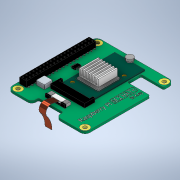
# Autodesk Inventor part: Raspberry Pi HAT+
Saved by Autodesk Inventor 2021 (Build 250183000, 183)
## iProperties
Created: 2025-01-26
Part Number: Raspberry Pi HAT+
Material: Generic
Document SubType Name: Modeling
Designer: 22liatho
Density: 1 g/cm^3
Appearance: Default
Author: 22liatho
Autodesk Inventor part; units mm, degrees
(part 1 of 2)
sketch "Sketch1" plane through (0, 0, 0) normal (0, 1, 0) x (-1, 0, 0)
  line L0 (-53, -65) -> (-3.5, -65)
  line L1 (0, -61.5) -> (0, -3.5)
  arc A0 (-3.5, -65) -> (0, -61.5) centre (-3.5, -61.5) ccw
  arc A1 (0, -3.5) -> (-3.5, 0) centre (-3.5, -3.5) ccw
  arc A2 (-53, 0) -> (-56.5, -3.5) centre (-53, -3.5) ccw
  arc A3 (-56.5, -61.5) -> (-53, -65) centre (-53, -61.5) ccw
  line L2 (-56.5, -57.5) -> (-40, -57.5)
  line L3 (-40, -57.5) -> (-40, -47.5)
  line L4 (-40, -47.5) -> (-56.5, -47.5)
  circle A4 centre (-53, -3.5) radius 3
  line L5 (-17.5, 0) -> (-17.5, -5)
  line L6 (-17.5, -5) -> (-35.5, -5)
  line L7 (-35.5, -5) -> (-35.5, 0)
  line L8 (-1.5, -7.1) -> (-6.5, -7.1)
  line L9 (-6.5, -7.1) -> (-6.5, -57.9)
  line L10 (-6.5, -57.9) -> (-1.5, -57.9)
  line L11 (-1.5, -57.9) -> (-1.5, -7.1)
  line L12 (-3.5, 0) -> (-17.5, 0)
  line L13 (-35.5, 0) -> (-53, 0)
  line L14 (-56.5, -3.5) -> (-56.5, -47.5)
  line L15 (-56.5, -57.5) -> (-56.5, -61.5)
  circle A5 centre (-53, -61.5) radius 3
  circle A6 centre (-53, -3.5) radius 1.375
  circle A7 centre (-53, -61.5) radius 1.375
  circle A8 centre (-4, -61.5) radius 3
  circle A9 centre (-4, -61.5) radius 1.375
  circle A10 centre (-4, -3.5) radius 3
  circle A11 centre (-4, -3.5) radius 1.375
  line L16 (-1.5, -32.5) -> (-6.5, -32.5) construction
  point P0 (0, 0)
  point P1 (-56.5, -65)
  point P2 (0, -65)
  point P3 (-4, -32.5)
  dimension "d82" = 3
  dimension "d83" = 3
  dimension "d2" = 3.5
  dimension "d5" = 7.5
  dimension "d6" = 10
  dimension "d10" = 18
  dimension "d12" = 17.5
  dimension "d17" = 5
  dimension "d18" = 56.5
  dimension "d19" = 16.5
  dimension "d20" = 65
  dimension "d21" = 3.5
  dimension "d22" = 3.5
  dimension "d23" = 58
  dimension "d24" = 3.5
  dimension "d25" = 6
  dimension "d26" = 6
  dimension "d27" = 2.75
  dimension "d28" = 2.75
  dimension "d29" = 3.5
  dimension "d31" = 6
  dimension "d32" = 2.75
  dimension "d35" = 49
  dimension "d36" = 6
  dimension "d37" = 49
  dimension "d38" = 3.5
  dimension "d39" = 2.75
  dimension "d40" = 29
  dimension "d43" = 5
  dimension "d44" = 56.5
  dimension "d206" = 50.8
  constraints: 34 end point, 12 centre point, 12 tangent, 10 perpendicular, 8 point on circle, 6 parallel, 5 horizontal, 4 coincident, 4 point on line, 3 equal radius, 3 midpoint, 1 horizontal alignment, 1 vertical, 1 vertical alignment
  measures "d2" radius of A0
  measures "d5" distance between parallel lines of L0 L2
  measures "d6" distance between parallel lines of L2 L4
  measures "d10" distance between parallel lines of L7 L5
  measures "d12" distance between parallel lines of L1 L5
  measures "d17" distance between parallel lines of L12 L6
  measures "d18" distance between parallel lines of L1 L14
  measures "d19" distance between parallel lines of L14 L3
  measures "d20" distance between parallel lines of L13 L0
  measures "d21" distance from line of L14 A4.centre
  measures "d22" distance from line of L13 A4.centre
  measures "d23" distance of A2.centre A5.centre
  measures "d24" distance from line of L15 A5.centre
  measures "d25" diameter of A4
  measures "d26" diameter of A5
  measures "d27" diameter of A6
  measures "d28" diameter of A7
  measures "d29" distance from line of L0 A8.centre
  measures "d31" diameter of A8
  measures "d32" diameter of A9
  measures "d35" distance of A5.centre A8.centre
  measures "d36" diameter of A10
  measures "d37" distance of A4.centre A10.centre
  measures "d38" distance from line of L12 A10.centre
  measures "d39" diameter of A11
  measures "d40" distance from line of A10.centre L16
  measures "d43" distance between parallel lines of L11 L9
  measures "d44" distance from line of point (-56.5, -65) L1
  measures "d206" distance of L10.end L8.start
extrude "Extrusion1" add sketch "Sketch1" along normal blind 1.6 contours A3 L15 L2 L3 L4 L14 A2 L13 L7 L6 L5 L12 A1 L1 A0 L0 | L11 L10 L9 L8
extrude "Extrusion2" add sketch "Sketch1" along normal blind 1.58 contours A4 | A5 | A8 | A10
extrude "Extrusion3" add sketch "Sketch1" along normal blind 5.88 contours L11 L10 L9 L8
fillet "Fillet1" radius 3 2 edges at (35.5, 0.8, 0) (17.5, 0.8, 0)
sketch "Sketch2" plane through (0, 5.88, 0) normal (0, 1, 0) x (1, 0, 0)
  line L0 (2.45, 8.69) -> (3.09, 8.69)
  line L1 (3.09, 8.69) -> (3.09, 8.05)
  line L2 (3.09, 8.05) -> (2.45, 8.05)
  line L3 (2.45, 8.05) -> (2.45, 8.69)
  line L4 (1.5, 57.9) -> (1.5, 7.1) projected
  line L5 (1.5, 7.1) -> (6.5, 7.1) projected
  line L6 (5.55, 8.69) -> (5.55, 8.05)
  line L7 (5.55, 8.05) -> (4.91, 8.05)
  line L8 (4.91, 8.05) -> (4.91, 8.69)
  line L9 (4.91, 8.69) -> (5.55, 8.69)
  line L10 (3.09, 11.23) -> (3.09, 10.59)
  line L11 (3.09, 10.59) -> (2.45, 10.59)
  line L12 (2.45, 10.59) -> (2.45, 11.23)
  line L13 (2.45, 11.23) -> (3.09, 11.23)
  line L14 (5.55, 11.23) -> (5.55, 10.59)
  line L15 (5.55, 10.59) -> (4.91, 10.59)
  line L16 (4.91, 10.59) -> (4.91, 11.23)
  line L17 (4.91, 11.23) -> (5.55, 11.23)
  line L18 (3.09, 13.77) -> (3.09, 13.13)
  line L19 (3.09, 13.13) -> (2.45, 13.13)
  line L20 (2.45, 13.13) -> (2.45, 13.77)
  line L21 (2.45, 13.77) -> (3.09, 13.77)
  line L22 (5.55, 13.77) -> (5.55, 13.13)
  line L23 (5.55, 13.13) -> (4.91, 13.13)
  line L24 (4.91, 13.13) -> (4.91, 13.77)
  line L25 (4.91, 13.77) -> (5.55, 13.77)
  line L26 (3.09, 16.31) -> (3.09, 15.67)
  line L27 (3.09, 15.67) -> (2.45, 15.67)
  line L28 (2.45, 15.67) -> (2.45, 16.31)
  line L29 (2.45, 16.31) -> (3.09, 16.31)
  line L30 (5.55, 16.31) -> (5.55, 15.67)
  line L31 (5.55, 15.67) -> (4.91, 15.67)
  line L32 (4.91, 15.67) -> (4.91, 16.31)
  line L33 (4.91, 16.31) -> (5.55, 16.31)
  line L34 (3.09, 18.85) -> (3.09, 18.21)
  line L35 (3.09, 18.21) -> (2.45, 18.21)
  line L36 (2.45, 18.21) -> (2.45, 18.85)
  line L37 (2.45, 18.85) -> (3.09, 18.85)
  line L38 (5.55, 18.85) -> (5.55, 18.21)
  line L39 (5.55, 18.21) -> (4.91, 18.21)
  line L40 (4.91, 18.21) -> (4.91, 18.85)
  line L41 (4.91, 18.85) -> (5.55, 18.85)
  line L42 (3.09, 21.39) -> (3.09, 20.75)
  line L43 (3.09, 20.75) -> (2.45, 20.75)
  line L44 (2.45, 20.75) -> (2.45, 21.39)
  line L45 (2.45, 21.39) -> (3.09, 21.39)
  line L46 (5.55, 21.39) -> (5.55, 20.75)
  line L47 (5.55, 20.75) -> (4.91, 20.75)
  line L48 (4.91, 20.75) -> (4.91, 21.39)
  line L49 (4.91, 21.39) -> (5.55, 21.39)
  line L50 (3.09, 23.93) -> (3.09, 23.29)
  line L51 (3.09, 23.29) -> (2.45, 23.29)
  line L52 (2.45, 23.29) -> (2.45, 23.93)
  line L53 (2.45, 23.93) -> (3.09, 23.93)
  line L54 (5.55, 23.93) -> (5.55, 23.29)
  line L55 (5.55, 23.29) -> (4.91, 23.29)
  line L56 (4.91, 23.29) -> (4.91, 23.93)
  line L57 (4.91, 23.93) -> (5.55, 23.93)
  line L58 (3.09, 26.47) -> (3.09, 25.83)
  line L59 (3.09, 25.83) -> (2.45, 25.83)
  line L60 (2.45, 25.83) -> (2.45, 26.47)
  line L61 (2.45, 26.47) -> (3.09, 26.47)
  line L62 (5.55, 26.47) -> (5.55, 25.83)
  line L63 (5.55, 25.83) -> (4.91, 25.83)
  line L64 (4.91, 25.83) -> (4.91, 26.47)
  line L65 (4.91, 26.47) -> (5.55, 26.47)
  line L66 (3.09, 29.01) -> (3.09, 28.37)
  line L67 (3.09, 28.37) -> (2.45, 28.37)
  line L68 (2.45, 28.37) -> (2.45, 29.01)
  line L69 (2.45, 29.01) -> (3.09, 29.01)
  line L70 (5.55, 29.01) -> (5.55, 28.37)
  line L71 (5.55, 28.37) -> (4.91, 28.37)
  line L72 (4.91, 28.37) -> (4.91, 29.01)
  line L73 (4.91, 29.01) -> (5.55, 29.01)
  line L74 (3.09, 31.55) -> (3.09, 30.91)
  line L75 (3.09, 30.91) -> (2.45, 30.91)
  line L76 (2.45, 30.91) -> (2.45, 31.55)
  line L77 (2.45, 31.55) -> (3.09, 31.55)
  line L78 (5.55, 31.55) -> (5.55, 30.91)
  line L79 (5.55, 30.91) -> (4.91, 30.91)
  line L80 (4.91, 30.91) -> (4.91, 31.55)
  line L81 (4.91, 31.55) -> (5.55, 31.55)
  line L82 (3.09, 34.09) -> (3.09, 33.45)
  line L83 (3.09, 33.45) -> (2.45, 33.45)
  line L84 (2.45, 33.45) -> (2.45, 34.09)
  line L85 (2.45, 34.09) -> (3.09, 34.09)
  line L86 (5.55, 34.09) -> (5.55, 33.45)
  line L87 (5.55, 33.45) -> (4.91, 33.45)
  line L88 (4.91, 33.45) -> (4.91, 34.09)
  line L89 (4.91, 34.09) -> (5.55, 34.09)
  line L90 (3.09, 36.63) -> (3.09, 35.99)
  line L91 (3.09, 35.99) -> (2.45, 35.99)
  line L92 (2.45, 35.99) -> (2.45, 36.63)
  line L93 (2.45, 36.63) -> (3.09, 36.63)
  line L94 (5.55, 36.63) -> (5.55, 35.99)
  line L95 (5.55, 35.99) -> (4.91, 35.99)
  line L96 (4.91, 35.99) -> (4.91, 36.63)
  line L97 (4.91, 36.63) -> (5.55, 36.63)
  line L98 (3.09, 39.17) -> (3.09, 38.53)
  line L99 (3.09, 38.53) -> (2.45, 38.53)
  line L100 (2.45, 38.53) -> (2.45, 39.17)
  line L101 (2.45, 39.17) -> (3.09, 39.17)
  line L102 (5.55, 39.17) -> (5.55, 38.53)
  line L103 (5.55, 38.53) -> (4.91, 38.53)
  line L104 (4.91, 38.53) -> (4.91, 39.17)
  line L105 (4.91, 39.17) -> (5.55, 39.17)
  line L106 (3.09, 41.71) -> (3.09, 41.07)
  line L107 (3.09, 41.07) -> (2.45, 41.07)
  line L108 (2.45, 41.07) -> (2.45, 41.71)
  line L109 (2.45, 41.71) -> (3.09, 41.71)
  line L110 (5.55, 41.71) -> (5.55, 41.07)
  line L111 (5.55, 41.07) -> (4.91, 41.07)
  line L112 (4.91, 41.07) -> (4.91, 41.71)
  line L113 (4.91, 41.71) -> (5.55, 41.71)
  line L114 (3.09, 44.25) -> (3.09, 43.61)
  line L115 (3.09, 43.61) -> (2.45, 43.61)
  line L116 (2.45, 43.61) -> (2.45, 44.25)
  line L117 (2.45, 44.25) -> (3.09, 44.25)
  line L118 (5.55, 44.25) -> (5.55, 43.61)
  line L119 (5.55, 43.61) -> (4.91, 43.61)
  line L120 (4.91, 43.61) -> (4.91, 44.25)
  line L121 (4.91, 44.25) -> (5.55, 44.25)
  line L122 (3.09, 46.79) -> (3.09, 46.15)
  line L123 (3.09, 46.15) -> (2.45, 46.15)
  line L124 (2.45, 46.15) -> (2.45, 46.79)
  line L125 (2.45, 46.79) -> (3.09, 46.79)
  line L126 (5.55, 46.79) -> (5.55, 46.15)
  line L127 (5.55, 46.15) -> (4.91, 46.15)
  line L128 (4.91, 46.15) -> (4.91, 46.79)
  line L129 (4.91, 46.79) -> (5.55, 46.79)
  line L130 (3.09, 49.33) -> (3.09, 48.69)
  line L131 (3.09, 48.69) -> (2.45, 48.69)
  line L132 (2.45, 48.69) -> (2.45, 49.33)
  line L133 (2.45, 49.33) -> (3.09, 49.33)
  line L134 (5.55, 49.33) -> (5.55, 48.69)
  line L135 (5.55, 48.69) -> (4.91, 48.69)
  line L136 (4.91, 48.69) -> (4.91, 49.33)
  line L137 (4.91, 49.33) -> (5.55, 49.33)
  line L138 (3.09, 51.87) -> (3.09, 51.23)
  line L139 (3.09, 51.23) -> (2.45, 51.23)
  line L140 (2.45, 51.23) -> (2.45, 51.87)
  line L141 (2.45, 51.87) -> (3.09, 51.87)
  line L142 (5.55, 51.87) -> (5.55, 51.23)
  line L143 (5.55, 51.23) -> (4.91, 51.23)
  line L144 (4.91, 51.23) -> (4.91, 51.87)
  line L145 (4.91, 51.87) -> (5.55, 51.87)
  line L146 (3.09, 54.41) -> (3.09, 53.77)
  line L147 (3.09, 53.77) -> (2.45, 53.77)
  line L148 (2.45, 53.77) -> (2.45, 54.41)
  line L149 (2.45, 54.41) -> (3.09, 54.41)
  line L150 (5.55, 54.41) -> (5.55, 53.77)
  line L151 (5.55, 53.77) -> (4.91, 53.77)
  line L152 (4.91, 53.77) -> (4.91, 54.41)
  line L153 (4.91, 54.41) -> (5.55, 54.41)
  line L154 (3.09, 56.95) -> (3.09, 56.31)
  line L155 (3.09, 56.31) -> (2.45, 56.31)
  line L156 (2.45, 56.31) -> (2.45, 56.95)
  line L157 (2.45, 56.95) -> (3.09, 56.95)
  line L158 (5.55, 56.95) -> (5.55, 56.31)
  line L159 (5.55, 56.31) -> (4.91, 56.31)
  line L160 (4.91, 56.31) -> (4.91, 56.95)
  line L161 (4.91, 56.95) -> (5.55, 56.95)
  line L162 (6.5, 57.9) -> (1.5, 57.9) projected
  point P0 (0, 0)
  dimension "d54" = 0.95
  dimension "d55" = 0.95
  dimension "d56" = 0.64
  dimension "d57" = 0.64
  dimension "d60" = 2.46
  dimension "d63" = 2.54
  dimension "d66" = 0.95
  constraints: 320 end point, 2 horizontal, 2 parallel, 1 perpendicular, 1 vertical, 312 other
  measures "d54" distance between parallel lines of L4 L3
  measures "d55" distance between parallel lines of L5 L2
  measures "d56" distance of L0.start L0.end
  measures "d57" distance of L0.end L1.end
  measures "d60" distance of L0.end L6.start
  measures "d63" distance of L0.end L10.start
  measures "d66" distance between parallel lines of L162 L157
extrude "Extrusion4" cut sketch "Sketch2" against normal blind 1
fillet "Fillet4" radius 1 6 edges at (40, 0.8, -57.5) (40, 0.8, -47.5) (56.5, 0.8, -47.5) (56.5, 0.8, -57.5) (17.5, 0.8, -5) (35.5, 0.8, -5)
sketch "Sketch3" plane through (0, 1.6, 0) normal (0, 1, 0) x (1, 0, 0)
  line L0 (17.25, 19) -> (39.25, 19)
  line L1 (39.25, 19) -> (39.25, 61)
  line L2 (39.25, 61) -> (17.25, 61)
  line L3 (17.25, 61) -> (17.25, 19)
  circle A0 centre (35.75, 49.5) radius 1.25
  circle A1 centre (20.75, 26.5) radius 1.25
  line L4 (53, 65) -> (3.5, 65) projected
  circle A2 centre (28.25, 61) radius 2
  line L5 (19.75, 29.5) -> (36.75, 29.5)
  line L6 (36.75, 29.5) -> (36.75, 46.5)
  line L7 (36.75, 46.5) -> (19.75, 46.5)
  line L8 (19.75, 46.5) -> (19.75, 29.5)
  line L9 (18.25, 19) -> (18.25, 22.5)
  line L10 (21.75, 19) -> (21.75, 22)
  arc A3 (22.75, 22) -> (21.75, 22) centre (22.25, 22) ccw
  line L11 (22.75, 22) -> (22.75, 19)
  line L12 (33.75, 19) -> (33.75, 22)
  arc A4 (34.75, 22) -> (33.75, 22) centre (34.25, 22) ccw
  line L13 (34.75, 22) -> (34.75, 19)
  line L14 (38.25, 19) -> (38.25, 22.5)
  line L15 (39.25, 23) -> (38.75, 23)
  arc A5 (38.75, 23) -> (38.25, 22.5) centre (38.75, 22.5) ccw
  line L16 (17.25, 23) -> (17.75, 23)
  arc A6 (18.25, 22.5) -> (17.75, 23) centre (17.75, 22.5) ccw
  point P0 (0, 0)
  point P1 (28.25, 65)
  point P2 (28.25, 46.5)
  point P3 (34.25, 22.5)
  point P4 (22.25, 22.5)
  point P5 (30.25, 61)
  point P6 (26.25, 61)
  dimension "d69" = 22
  dimension "d70" = 42
  dimension "d71" = 2.5
  dimension "d72" = 2.5
  dimension "d73" = 18.5
  dimension "d74" = 3.5
  dimension "d75" = 30.5
  dimension "d76" = 7.5
  dimension "d78" = 4
  dimension "d79" = 17
  dimension "d80" = 17
  dimension "d81" = 4
  dimension "d82" = 3
  dimension "d83" = 3
  dimension "d84" = 1
  dimension "d85" = 1
  dimension "d86" = 0.5
  dimension "d87" = 4
  dimension "d88" = 1
  dimension "d89" = 1
  dimension "d90" = 4.5
  dimension "d91" = 4.5
  dimension "d92" = 0.5
  dimension "d93" = 4
  dimension "d94" = 3.5
  dimension "d95" = 3.5
  constraints: 32 end point, 10 point on circle, 8 point on line, 8 tangent, 7 centre point, 5 perpendicular, 4 parallel, 4 vertical, 3 horizontal, 3 midpoint, 2 vertical alignment, 1 coincident
  measures "d69" distance of L1.end L2.end
  measures "d70" distance of L0.end L1.end
  measures "d71" diameter of A0
  measures "d72" diameter of A1
  measures "d73" distance from line of L1 A1.centre
  measures "d74" distance from line of L1 A0.centre
  measures "d75" distance from line of L0 A0.centre
  measures "d76" distance from line of L0 A1.centre
  measures "d78" distance between parallel lines of L4 L2
  measures "d79" distance of L6.end L7.end
  measures "d80" distance of L7.end L5.start
  measures "d81" diameter of A2
  measures "d82" distance from line of A0.centre L7
  measures "d83" distance from line of A1.centre L5
  measures "d84" distance between parallel lines of L1 L14
  measures "d85" distance between parallel lines of L3 L9
  measures "d86" distance of L15.start L15.end
  measures "d87" distance of L0.end L15.start
  measures "d88" distance between parallel lines of L12 L13
  measures "d89" distance between parallel lines of L11 L10
  measures "d90" distance between parallel lines of L1 L13
  measures "d91" distance between parallel lines of L3 L10
  measures "d92" distance of L16.start L16.end
  measures "d93" distance between parallel lines of L0 L16
  measures "d94" distance from line of L0 point (34.25, 22.5)
  measures "d95" distance from line of L0 point (22.25, 22.5)
extrude "Extrusion5" add sketch "Sketch3" along normal blind 1 contours L9 A6 L16 L3 L2 A2 L1 L15 A5 L14 L0 L13 A4 L12 L11 A3 L10 | L8 L7 L6 L5
sketch "Sketch4" plane through (0, 1.6, 0) normal (0, 1, 0) x (1, 0, 0)
  circle A0 centre (28.25, 61) radius 2
  arc A1 (26.25, 61) -> (30.25, 61) centre (28.25, 61) ccw projected
  line L0 (26.25, 61) -> (17.25, 61) projected
  line L1 (39.25, 61) -> (30.25, 61) projected
  point P0 (0, 0)
  dimension "d98" = 4
  constraints: 1 centre point, 1 coincident, 1 horizontal alignment
  measures "d98" diameter of A0
extrude "Extrusion6" cut sketch "Sketch4" against normal through all
extrude "Extrusion7" add sketch "Sketch3" along normal blind 1.25 contours L8 L7 L6 L5
sketch "Sketch5" plane through (0, 2.85, 0) normal (0, 1, 0) x (1, 0, 0)
  line L0 (21, 30) -> (35.5, 30)
  line L1 (36.25, 30.75) -> (36.25, 45.25)
  line L2 (35.5, 46) -> (21, 46)
  line L3 (20.25, 45.25) -> (20.25, 30.75)
  line L4 (36.75, 46.5) -> (19.75, 46.5) projected
  line L5 (36.75, 29.5) -> (36.75, 46.5) projected
  line L6 (19.75, 29.5) -> (36.75, 29.5) projected
  line L7 (19.75, 46.5) -> (19.75, 29.5) projected
  arc A0 (20.25, 30.75) -> (21, 30) centre (21, 30.75) ccw
  arc A1 (35.5, 30) -> (36.25, 30.75) centre (35.5, 30.75) ccw
  arc A2 (36.25, 45.25) -> (35.5, 46) centre (35.5, 45.25) ccw
  arc A3 (21, 46) -> (20.25, 45.25) centre (21, 45.25) ccw
  point P0 (0, 0)
  dimension "d103" = 0.5
  dimension "d104" = 0.5
  dimension "d105" = 0.5
  dimension "d106" = 0.5
  dimension "d107" = 0.75
  constraints: 8 end point, 8 point on circle, 8 tangent, 4 centre point, 3 equal radius, 2 parallel, 1 horizontal, 1 perpendicular
  measures "d103" distance between parallel lines of L4 L2
  measures "d104" distance between parallel lines of L5 L1
  measures "d105" distance between parallel lines of L6 L0
  measures "d106" distance between parallel lines of L7 L3
  measures "d107" radius of A0
extrude "Extrusion8" add sketch "Sketch5" along normal blind 0.5 contours A0 L3 A3 L2 A2 L1 A1 L0
sketch "Sketch6" plane through (0, 3.35, 0) normal (0, 1, 0) x (1, 0, 0)
  line L0 (23.75, 32.5) -> (32.75, 32.5)
  line L1 (33.75, 33.5) -> (33.75, 42.5)
  line L2 (32.75, 43.5) -> (23.75, 43.5)
  line L3 (22.75, 42.5) -> (22.75, 33.5)
  line L4 (21, 30) -> (35.5, 30) projected
  line L5 (20.25, 45.25) -> (20.25, 30.75) projected
  line L6 (35.5, 46) -> (21, 46) projected
  line L7 (36.25, 30.75) -> (36.25, 45.25) projected
  arc A0 (33.75, 42.5) -> (32.75, 43.5) centre (32.75, 42.5) ccw
  arc A1 (32.75, 32.5) -> (33.75, 33.5) centre (32.75, 33.5) ccw
  arc A2 (22.75, 33.5) -> (23.75, 32.5) centre (23.75, 33.5) ccw
  arc A3 (23.75, 43.5) -> (22.75, 42.5) centre (23.75, 42.5) ccw
  point P0 (0, 0)
  dimension "d110" = 2.5
  dimension "d111" = 2.5
  dimension "d112" = 2.5
  dimension "d113" = 2.5
  dimension "d114" = 1
  constraints: 8 end point, 8 point on circle, 8 tangent, 4 centre point, 3 equal radius, 2 parallel, 1 horizontal, 1 perpendicular
  measures "d110" distance between parallel lines of L4 L0
  measures "d111" distance between parallel lines of L5 L3
  measures "d112" distance between parallel lines of L6 L2
  measures "d113" distance between parallel lines of L1 L7
  measures "d114" radius of A0
extrude "Extrusion9" add sketch "Sketch6" along normal blind 1
chamfer "Chamfer1" distance 0.5 distance2 1 8 edges at (33.75, 4.35, -38) (33.4571, 4.35, -43.2071) (28.25, 4.35, -43.5) (23.0429, 4.35, -43.2071) (22.75, 4.35, -38) (23.0429, 4.35, -32.7929) (28.25, 4.35, -32.5) (33.4571, 4.35, -32.7929) measured on face at (28.25, 4.35, -33) measured on face at (28.25, 4.35, -43) measured on face at (23.3964, 4.35, -33.1464) measured on face at (33.1036, 4.35, -33.1464) measured on face at (23.3964, 4.35, -42.8536) measured on face at (23.25, 4.35, -38) measured on face at (33.1036, 4.35, -42.8536) measured on face at (33.25, 4.35, -38)
fillet "Fillet6" radius 0.25 8 edges at (33.1036, 4.35, -33.1464) (28.25, 4.35, -32.9999) (23.3964, 4.35, -33.1464) (23.2499, 4.35, -38) (23.3964, 4.35, -42.8536) (28.25, 4.35, -43.0001) (33.1036, 4.35, -42.8536) (33.2501, 4.35, -38)
sketch "Sketch7" plane through (0, 1.6, 0) normal (0, 1, 0) x (1, 0, 0)
  circle A0 centre (28.25, 61) radius 2
  arc A1 (30.25, 61) -> (26.25, 61) centre (28.25, 61) ccw projected
  point P0 (0, 0)
  constraints: 1 coincident, 1 horizontal alignment, 2 other
extrude "Extrusion10" add sketch "Sketch7" along normal blind 2 and the other way blind 1.6
sketch "Sketch8" plane through (28.25, 3.6, -61) normal (0, 1, 0) x (1, 0, 0)
  circle A0 centre (0, 0) radius 2.5
  circle A1 centre (0, 0) radius 2 projected
  circle A2 centre (0, 2.5) radius 0.125
  circle A3 centre (-1.0168, 2.2839) radius 0.125
  circle A4 centre (-1.8579, 1.6728) radius 0.125
  circle A5 centre (-2.3776, 0.7725) radius 0.125
  circle A6 centre (-2.4863, -0.2613) radius 0.125
  circle A7 centre (-2.1651, -1.25) radius 0.125
  circle A8 centre (-1.4695, -2.0225) radius 0.125
  circle A9 centre (-0.5198, -2.4454) radius 0.125
  circle A10 centre (0.5198, -2.4454) radius 0.125
  circle A11 centre (1.4695, -2.0225) radius 0.125
  circle A12 centre (2.1651, -1.25) radius 0.125
  circle A13 centre (2.4863, -0.2613) radius 0.125
  circle A14 centre (2.3776, 0.7725) radius 0.125
  circle A15 centre (1.8579, 1.6728) radius 0.125
  circle A16 centre (1.0168, 2.2839) radius 0.125
  point P0 (-28.25, -61)
  point P1 (1.1297, 2.2302)
  point P2 (0.9014, 2.3318)
  point P3 (0.125, 2.4969)
  point P4 (-0.125, 2.4969)
  point P5 (-0.9014, 2.3318)
  point P6 (-1.1297, 2.2302)
  point P7 (-1.7719, 1.7636)
  point P8 (-1.9392, 1.5779)
  point P9 (-2.3361, 0.8904)
  point P10 (-2.4133, 0.6527)
  point P11 (-2.4963, -0.1367)
  point P12 (-2.4701, -0.3853)
  point P13 (-2.2248, -1.1402)
  point P14 (-2.0999, -1.3567)
  point P15 (-1.5687, -1.9466)
  point P16 (-1.3665, -2.0935)
  point P17 (-0.6414, -2.4163)
  point P18 (-0.3969, -2.4683)
  point P19 (0.3969, -2.4683)
  point P20 (0.6414, -2.4163)
  point P21 (1.3665, -2.0935)
  point P22 (1.5687, -1.9466)
  point P23 (2.0999, -1.3567)
  point P24 (2.2248, -1.1402)
  point P25 (2.4701, -0.3853)
  point P26 (2.4963, -0.1367)
  point P27 (2.4133, 0.6527)
  point P28 (2.3361, 0.8904)
  point P29 (1.9392, 1.5779)
  point P30 (1.7719, 1.7636)
  dimension "d126" = 5
  dimension "d127" = 0.25
  dimension "d130" = 360
  constraints: 15 centre point, 1 coincident, 34 other
  measures "d127" diameter of A2
extrude "Extrusion11" add sketch "Sketch8" along normal blind 1.5 contours A0 A13 A12 A11 A10 A9 A8 A7 A6 A5 A4 A3 A2 A16 A15 A14 | A1
sketch "Sketch9" plane through (0, 1.6, 0) normal (0, 1, 0) x (1, 0, 0)
  line L0 (15.75, 23) -> (17.25, 23)
  line L1 (17.25, 23) -> (17.25, 17)
  line L2 (17.25, 17) -> (15.75, 17)
  line L3 (15.75, 17) -> (15.75, 23)
  line L4 (15.75, 17) -> (40.75, 17)
  line L5 (40.75, 17) -> (40.75, 15.5)
  line L6 (40.75, 15.5) -> (15.75, 15.5)
  line L7 (15.75, 15.5) -> (15.75, 17)
  line L8 (40.75, 17) -> (39.25, 17)
  line L9 (39.25, 17) -> (39.25, 23)
  line L10 (39.25, 23) -> (40.75, 23)
  line L11 (40.75, 23) -> (40.75, 17)
  line L12 (38.25, 19) -> (38.25, 22.5) projected
  line L13 (18.25, 22.5) -> (18.25, 19) projected
  line L14 (22.75, 19) -> (33.75, 19) projected
  point P0 (0, 0)
  point P1 (39.25, 23)
  point P2 (17.25, 23)
  dimension "d134" = 1.5
  dimension "d135" = 1.5
  dimension "d136" = 1
  dimension "d137" = 1
  dimension "d138" = 1.5
  dimension "d139" = 2
  constraints: 24 end point, 6 parallel, 3 horizontal, 3 perpendicular, 2 coincident
  measures "d134" distance between parallel lines of L11 L9
  measures "d135" distance between parallel lines of L3 L1
  measures "d136" distance between parallel lines of L12 L9
  measures "d137" distance between parallel lines of L1 L13
  measures "d138" distance between parallel lines of L6 L4
  measures "d139" distance between parallel lines of L14 L4
extrude "Extrusion12" add sketch "Sketch9" along normal blind 3
sketch "Sketch10" plane through (39.25, 1.6, -17) normal (0, 0, -1) x (-1, 0, 0)
  line L0 (22, 0) -> (22, 3) projected
  line L1 (0, 3) -> (22, 3)
  line L2 (22, 3) -> (22, 2.25)
  line L3 (22, 2.25) -> (0, 2.25)
  line L4 (0, 2.25) -> (0, 3)
  point P0 (39.25, -1.6)
  dimension "d142" = 0.75
  constraints: 8 end point, 2 parallel, 1 horizontal, 1 perpendicular, 1 point on line
  measures "d142" distance between parallel lines of L1 L3
extrude "Extrusion13" add sketch "Sketch10" along normal blind 3.5
sketch "Sketch11" plane through (0, 1.6, 0) normal (0, 1, 0) x (1, 0, 0)
  line L0 (19.5, 12.5) -> (33.5, 12.5)
  line L1 (33.5, 12.5) -> (33.5, 9)
  line L2 (33.5, 9) -> (19.5, 9)
  line L3 (19.5, 9) -> (19.5, 12.5)
  line L4 (35.5, 4) -> (35.5, 3) projected
  line L5 (17.5, 3) -> (17.5, 4) projected
  line L6 (18.5, 5) -> (34.5, 5) projected
  line L7 (30.5, 9) -> (30.5, 12.5)
  line L8 (22.5, 9) -> (22.5, 12.5)
  point P0 (0, 0)
  dimension "d145" = 2
  dimension "d146" = 2
  dimension "d147" = 4
  dimension "d148" = 3.5
  dimension "d207" = 3
  dimension "d208" = 3
  constraints: 12 end point, 4 point on line, 3 perpendicular, 2 parallel, 1 horizontal
  measures "d145" distance between parallel lines of L4 L1
  measures "d146" distance between parallel lines of L5 L3
  measures "d147" distance between parallel lines of L6 L2
  measures "d148" distance between parallel lines of L0 L2
  measures "d207" distance between parallel lines of L3 L8
  measures "d208" distance between parallel lines of L1 L7
extrude "Extrusion14" add sketch "Sketch11" along normal blind 2 contours L0 L8 L2 L3 | L0 L1 L2 L7
sketch "Sketch12" plane through (19.5, 1.6, -9) normal (0, 0, 1) x (1, 0, 0)
  line L0 (14, 0) -> (11, 0) projected
  line L1 (14, 0) -> (14, 2) projected
  line L2 (0, 2) -> (3, 2) projected
  line L3 (0, 0) -> (0, 2) projected
  line L4 (3.05, 0.5) -> (10.95, 0.5)
  line L5 (14, 2) -> (0, 2) projected
  line L6 (0, 2) -> (14, 2) projected
  line L7 (0, 2) -> (0, 2.25)
  line L8 (14, 0) -> (14, 2) projected
  line L9 (13.8191, 2.6118) -> (14.25, 1.75) projected
  line L10 (11.0026, 3.5) -> (11.0026, 2) projected
  line L11 (10.95, 2.25) -> (14.25, 2.25)
  line L12 (14.25, 2.25) -> (14.25, 0)
  line L13 (3.05, 2.25) -> (-0.25, 2.25)
  line L14 (-0.25, 2.25) -> (-0.25, 0)
  line L15 (0, 0) -> (3, 0) projected
  line L16 (14, 0) -> (11, 0) projected
  line L17 (-3.75, 0) -> (-2.25, 0) projected
  line L18 (-2.25, 0) -> (6.75, 0) projected
  line L19 (6.75, 0) -> (10.75, 0) projected
  line L20 (10.75, 0) -> (19.75, 0) projected
  line L21 (19.75, 0) -> (21.25, 0) projected
  line L22 (21.25, 0) -> (-3.75, 0) projected
  line L23 (37, 0) -> (36, 0) projected
  line L24 (37, 0) -> (33.5, 0) projected
  line L25 (33.5, 0) -> (-16, 0) projected
  line L26 (-16, 0) -> (-19.5, 0) projected
  line L27 (-19.5, 0) -> (-16, 0) projected
  line L28 (-16, 0) -> (-5, 0) projected
  line L29 (-2, 0) -> (-5, 0) projected
  line L30 (-1, 0) -> (-2, 0) projected
  line L31 (-1, 0) -> (15, 0) projected
  line L32 (16, 0) -> (15, 0) projected
  line L33 (19, 0) -> (16, 0) projected
  line L34 (19, 0) -> (33.5, 0) projected
  line L35 (33.5, 0) -> (37, 0) projected
  line L36 (36, 0) -> (37, 0) projected
  line L37 (36, 0) -> (21.5, 0) projected
  line L38 (20.5, 0) -> (21.5, 0) projected
  line L39 (21.5, 0) -> (20.5, 0) projected
  line L40 (21.5, 0) -> (36, 0) projected
  line L41 (-13, 0) -> (-18, 0) projected
  line L42 (-18, 0) -> (-13, 0) projected
  line L43 (-18.5, 0) -> (-12.5, 0) projected
  line L44 (-18.5, 0) -> (-12.5, 0) projected
  line L45 (30.5, 0) -> (36.5, 0) projected
  line L46 (30.5, 0) -> (36.5, 0) projected
  line L47 (11, 0) -> (14, 0) projected
  line L48 (3, 0) -> (0, 0) projected
  line L49 (11, 2) -> (14, 2) projected
  line L50 (11, 0) -> (11, 2) projected
  line L51 (3, 0) -> (0, 0) projected
  line L52 (3, 0) -> (3, 2) projected
  line L53 (3.05, 2.25) -> (3.05, 0.5)
  line L54 (10.95, 0.5) -> (10.95, 2.25)
  line L55 (-0.25, 0) -> (14.25, 0)
  point P0 (-19.5, -1.6)
  point P1 (3, 2)
  point P2 (14.25, 0)
  point P3 (11.0026, 2.25)
  point P4 (3, 0.5)
  point P5 (11, 0.5)
  point P6 (0, 0)
  dimension "d153" = 0.5
  dimension "d157" = 0.25
  dimension "d159" = 3.3
  dimension "d160" = 2.25
  dimension "d161" = 3.3
  dimension "d162" = 2.25
  dimension "d163" = 0.25
  dimension "d164" = 0.25
  constraints: 18 end point, 3 point on line, 3 vertical, 2 horizontal, 2 perpendicular, 1 collinear
  measures "d153" distance between parallel lines of L4 L0
  measures "d157" distance of L2.start L7.end
  measures "d159" distance of L11.start L11.end
  measures "d160" distance of L11.end L12.end
  measures "d161" distance of L13.start L13.end
  measures "d162" distance of L13.end L14.end
  measures "d163" distance between parallel lines of L1 L12
  measures "d164" distance between parallel lines of L14 L3
extrude "Extrusion15" add sketch "Sketch12" along normal blind 1 contours L0 L50 L5 L1 | L1 L5 L10 L11 L9 L12 L20 | L20 L19 L18 L52 L5 L53 L4 L54 L50 | L5 L54 L11 L10 | L9 L11 L12 | L15 L3 L2 L52 | L5 L2 L7 L13 L53 | L18 L14 L13 L7 L3
sketch "Sketch13" plane through (0, 1.6, 0) normal (0, 1, 0) x (1, 0, 0)
  line L0 (8.5, 18.5) -> (14, 18.5)
  line L1 (14.25, 18.25) -> (14.25, 12.75)
  line L2 (14, 12.5) -> (8.5, 12.5)
  line L3 (8.25, 12.75) -> (8.25, 18.25)
  line L4 (15.75, 23) -> (15.75, 15.5) projected
  line L5 (15.75, 15.5) -> (40.75, 15.5) projected
  arc A0 (8.25, 12.75) -> (8.5, 12.5) centre (8.5, 12.75) ccw
  arc A1 (8.5, 18.5) -> (8.25, 18.25) centre (8.5, 18.25) ccw
  arc A2 (14.25, 18.25) -> (14, 18.5) centre (14, 18.25) ccw
  arc A3 (14, 12.5) -> (14.25, 12.75) centre (14, 12.75) ccw
  point P0 (0, 0)
  point P1 (8.25, 18.5)
  point P2 (14.25, 12.5)
  point P3 (8.25, 12.5)
  dimension "d63" = 2.54
  dimension "d165" = 6
  dimension "d166" = 6
  dimension "d167" = 1.5
  dimension "d168" = 3
  dimension "d169" = 0.25
  constraints: 8 end point, 8 point on circle, 8 tangent, 6 point on line, 4 centre point, 3 equal radius, 2 parallel, 1 horizontal, 1 perpendicular
  measures "d165" distance of point (14.25, 12.5) point (8.25, 12.5)
  measures "d166" distance of point (8.25, 12.5) point (8.25, 18.5)
  measures "d167" distance between parallel lines of L4 L1
  measures "d168" distance between parallel lines of L2 L5
  measures "d169" radius of A0
extrude "Extrusion16" add sketch "Sketch13" along normal blind 3
sketch "Sketch14" plane through (0, 1.6, 0) normal (0, 1, 0) x (1, 0, 0)
  line L0 (41.6026, 4.6174) -> (41.6026, 28.8613) construction
  line L1 (41.6026, 28.8613) -> (53.1309, 28.8613) construction
  line L2 (53.1309, 28.8613) -> (53.1309, 4.6174) construction
  line L3 (53.1309, 4.6174) -> (41.6026, 4.6174) construction
  line L4 (39.9393, 25.3139) -> (39.9393, 50.4503) construction
  line L5 (39.9393, 50.4503) -> (53.8239, 50.4503) construction
  line L6 (53.8239, 50.4503) -> (53.8239, 25.3139) construction
  line L7 (53.8239, 25.3139) -> (39.9393, 25.3139) construction
  line L8 (50.1004, 38.4137) -> (50.1004, 53.4546) construction
  line L9 (50.1004, 53.4546) -> (55.1872, 53.4546) construction
  line L10 (55.1872, 53.4546) -> (55.1872, 38.4137) construction
  line L11 (55.1872, 38.4137) -> (50.1004, 38.4137) construction
  line L12 (48.5191, 7.9472) -> (48.5191, 7.4294)
  line L13 (48.5191, 7.4294) -> (47.3254, 6.4812)
  line L14 (47.3254, 6.4812) -> (47.3254, 6.0242)
  line L15 (47.3254, 6.0242) -> (48.5191, 6.0242)
  line L16 (48.5191, 6.0242) -> (48.5191, 5.6255)
  line L17 (48.5191, 5.6255) -> (45.5191, 5.6255)
  line L18 (45.5191, 5.6255) -> (45.5191, 6.3986)
  spline S0 degree 2 poles (45.5191, 6.3986) (45.5191, 6.6563) (45.575, 7.0039) (45.6771, 7.1619) knots 0 0 0 1 2 2 2
  spline S1 degree 2 poles (45.6771, 7.1619) (45.7792, 7.32) (46.0977, 7.5023) (46.3335, 7.5023) knots 0 0 0 1 2 2 2
  spline S2 degree 2 poles (46.3335, 7.5023) (46.6617, 7.5023) (47.1066, 7.1668) (47.2136, 6.8799) knots 0 0 0 1 2 2 2
  line L19 (47.2136, 6.8799) -> (48.5191, 7.9472)
  spline S3 degree 2 poles (46.3651, 7.0866) (46.2338, 7.0866) (46.0321, 6.9942) (45.9664, 6.8969) knots 0 0 0 1 2 2 2
  spline S4 degree 2 poles (45.9664, 6.8969) (45.9105, 6.8119) (45.8643, 6.5858) (45.8643, 6.4204) knots 0 0 0 1 2 2 2
  line L20 (45.8643, 6.4204) -> (45.8643, 6.0242)
  line L21 (45.8643, 6.0242) -> (46.9923, 6.0242)
  line L22 (46.9923, 6.0242) -> (46.9923, 6.3743)
  spline S5 degree 2 poles (46.9923, 6.3743) (46.9923, 6.5469) (46.9316, 6.8216) (46.8368, 6.9164) knots 0 0 0 1 2 2 2
  spline S6 degree 2 poles (46.8368, 6.9164) (46.7541, 7.0039) (46.5207, 7.0866) (46.3651, 7.0866) knots 0 0 0 1 2 2 2
  spline S7 degree 2 poles (48.2808, 9.4107) (48.3149, 9.3645) (48.4364, 9.2089) (48.4729, 9.136) knots 0 0 0 1 2 2 2
  spline S8 degree 2 poles (48.4729, 9.136) (48.5264, 9.0363) (48.5823, 8.8491) (48.5823, 8.679) knots 0 0 0 1 2 2 2
  spline S9 degree 2 poles (48.5823, 8.679) (48.5823, 8.5404) (48.4778, 8.29) (48.3829, 8.1952) knots 0 0 0 1 2 2 2
  spline S10 degree 2 poles (48.3829, 8.1952) (48.2906, 8.1052) (48.0183, 7.9958) (47.8676, 7.9958) knots 0 0 0 1 2 2 2
  spline S11 degree 2 poles (47.8676, 7.9958) (47.6342, 7.9958) (47.3035, 8.1927) (47.2087, 8.4067) knots 0 0 0 1 2 2 2
  spline S12 degree 2 poles (47.2087, 8.4067) (47.1212, 8.5963) (47.0556, 9.1117) (47.0385, 9.4107) knots 0 0 0 1 2 2 2
  line L23 (47.0385, 9.4107) -> (46.9656, 9.4107)
  spline S13 degree 2 poles (46.9656, 9.4107) (46.8343, 9.4107) (46.6714, 9.3305) (46.6253, 9.2576) knots 0 0 0 1 2 2 2
  spline S14 degree 2 poles (46.6253, 9.2576) (46.5791, 9.1846) (46.5499, 8.9756) (46.5499, 8.8637) knots 0 0 0 1 2 2 2
  spline S15 degree 2 poles (46.5499, 8.8637) (46.5499, 8.7324) (46.6277, 8.3775) (46.703, 8.2) knots 0 0 0 1 2 2 2
  line L24 (46.703, 8.2) -> (46.703, 8.1781)
  line L25 (46.703, 8.1781) -> (46.3165, 8.1781)
  spline S16 degree 2 poles (46.3165, 8.1781) (46.2873, 8.2827) (46.2144, 8.6741) (46.2144, 8.8662) knots 0 0 0 1 2 2 2
  spline S17 degree 2 poles (46.2144, 8.8662) (46.2144, 9.0995) (46.2873, 9.418) (46.3821, 9.5444) knots 0 0 0 1 2 2 2
  spline S18 degree 2 poles (46.3821, 9.5444) (46.4745, 9.6684) (46.7687, 9.79) (46.9802, 9.79) knots 0 0 0 1 2 2 2
  line L26 (46.9802, 9.79) -> (48.5191, 9.79)
  line L27 (48.5191, 9.79) -> (48.5191, 9.4107)
  line L28 (48.5191, 9.4107) -> (48.2808, 9.4107)
  line L29 (47.9648, 9.4107) -> (47.34, 9.4107)
  spline S19 degree 2 poles (47.34, 9.4107) (47.3522, 9.2746) (47.3935, 8.8637) (47.4324, 8.7349) knots 0 0 0 1 2 2 2
  spline S20 degree 2 poles (47.4324, 8.7349) (47.4786, 8.5841) (47.6706, 8.3872) (47.8408, 8.3872) knots 0 0 0 1 2 2 2
  spline S21 degree 2 poles (47.8408, 8.3872) (48.0353, 8.3872) (48.2322, 8.606) (48.2322, 8.8151) knots 0 0 0 1 2 2 2
  spline S22 degree 2 poles (48.2322, 8.8151) (48.2322, 8.9926) (48.0791, 9.2843) (47.9648, 9.4107) knots 0 0 0 1 2 2 2
  spline S23 degree 2 poles (48.5726, 10.9302) (48.5726, 10.7041) (48.451, 10.3127) (48.3829, 10.1838) knots 0 0 0 1 2 2 2
  line L30 (48.3829, 10.1838) -> (47.9575, 10.1838)
  line L31 (47.9575, 10.1838) -> (47.9575, 10.2033)
  spline S24 degree 2 poles (47.9575, 10.2033) (47.9964, 10.2519) (48.0888, 10.3832) (48.1398, 10.4926) knots 0 0 0 1 2 2 2
  spline S25 degree 2 poles (48.1398, 10.4926) (48.186, 10.5874) (48.2541, 10.8208) (48.2541, 10.9448) knots 0 0 0 1 2 2 2
  spline S26 degree 2 poles (48.2541, 10.9448) (48.2541, 11.0347) (48.2128, 11.2414) (48.1787, 11.29) knots 0 0 0 1 2 2 2
  spline S27 degree 2 poles (48.1787, 11.29) (48.1325, 11.3605) (48.028, 11.4237) (47.921, 11.4237) knots 0 0 0 1 2 2 2
  spline S28 degree 2 poles (47.921, 11.4237) (47.7873, 11.4237) (47.6488, 11.2778) (47.6026, 11.0906) knots 0 0 0 1 2 2 2
  spline S29 degree 2 poles (47.6026, 11.0906) (47.5855, 11.0177) (47.5369, 10.7843) (47.5102, 10.6846) knots 0 0 0 1 2 2 2
  spline S30 degree 2 poles (47.5102, 10.6846) (47.4348, 10.4269) (47.1236, 10.1935) (46.9024, 10.1935) knots 0 0 0 1 2 2 2
  spline S31 degree 2 poles (46.9024, 10.1935) (46.5961, 10.1935) (46.2144, 10.653) (46.2144, 11.0323) knots 0 0 0 1 2 2 2
  spline S32 degree 2 poles (46.2144, 11.0323) (46.2144, 11.2195) (46.3068, 11.5987) (46.3773, 11.7276) knots 0 0 0 1 2 2 2
  line L32 (46.3773, 11.7276) -> (46.7833, 11.7276)
  line L33 (46.7833, 11.7276) -> (46.7833, 11.7081)
  spline S33 degree 2 poles (46.7833, 11.7081) (46.6666, 11.5623) (46.5329, 11.2073) (46.5329, 11.025) knots 0 0 0 1 2 2 2
  spline S34 degree 2 poles (46.5329, 11.025) (46.5329, 10.8378) (46.6909, 10.5801) (46.8489, 10.5801) knots 0 0 0 1 2 2 2
  spline S35 degree 2 poles (46.8489, 10.5801) (46.9923, 10.5801) (47.1309, 10.7332) (47.1747, 10.9034) knots 0 0 0 1 2 2 2
  spline S36 degree 2 poles (47.1747, 10.9034) (47.1966, 10.9861) (47.2403, 11.1952) (47.2671, 11.3094) knots 0 0 0 1 2 2 2
  spline S37 degree 2 poles (47.2671, 11.3094) (47.3303, 11.5574) (47.6196, 11.8102) (47.87, 11.8102) knots 0 0 0 1 2 2 2
  spline S38 degree 2 poles (47.87, 11.8102) (48.0159, 11.8102) (48.2735, 11.696) (48.3684, 11.5841) knots 0 0 0 1 2 2 2
  spline S39 degree 2 poles (48.3684, 11.5841) (48.468, 11.465) (48.5726, 11.1611) (48.5726, 10.9302) knots 0 0 0 1 2 2 2
  spline S40 degree 2 poles (47.3327, 14.0493) (47.8967, 14.0493) (48.5629, 13.512) (48.5629, 13.1012) knots 0 0 0 1 2 2 2
  spline S41 degree 2 poles (48.5629, 13.1012) (48.5629, 12.9334) (48.4851, 12.6757) (48.4048, 12.542) knots 0 0 0 1 2 2 2
  line L34 (48.4048, 12.542) -> (49.3481, 12.542)
  line L35 (49.3481, 12.542) -> (49.3481, 12.1627)
  line L36 (49.3481, 12.1627) -> (46.2679, 12.1627)
  line L37 (46.2679, 12.1627) -> (46.2679, 12.542)
  line L38 (46.2679, 12.542) -> (46.5037, 12.542)
  spline S42 degree 2 poles (46.5037, 12.542) (46.3748, 12.683) (46.2047, 13.0282) (46.2047, 13.23) knots 0 0 0 1 2 2 2
  spline S43 degree 2 poles (46.2047, 13.23) (46.2047, 13.6166) (46.8173, 14.0493) (47.3327, 14.0493) knots 0 0 0 1 2 2 2
  spline S44 degree 2 poles (47.3765, 13.6579) (46.9899, 13.6579) (46.5645, 13.4123) (46.5645, 13.1376) knots 0 0 0 1 2 2 2
  spline S45 degree 2 poles (46.5645, 13.1376) (46.5645, 12.9772) (46.7079, 12.6757) (46.8197, 12.542) knots 0 0 0 1 2 2 2
  line L39 (46.8197, 12.542) -> (48.0985, 12.542)
  spline S46 degree 2 poles (48.0985, 12.542) (48.169, 12.6903) (48.2225, 12.9018) (48.2225, 13.0379) knots 0 0 0 1 2 2 2
  spline S47 degree 2 poles (48.2225, 13.0379) (48.2225, 13.3321) (47.7898, 13.6579) (47.3765, 13.6579) knots 0 0 0 1 2 2 2
  spline S48 degree 2 poles (47.357, 16.3297) (47.9089, 16.3297) (48.5823, 15.7948) (48.5823, 15.3913) knots 0 0 0 1 2 2 2
  spline S49 degree 2 poles (48.5823, 15.3913) (48.5823, 15.2089) (48.4923, 14.9488) (48.4146, 14.8224) knots 0 0 0 1 2 2 2
  line L40 (48.4146, 14.8224) -> (48.5191, 14.7981)
  line L41 (48.5191, 14.7981) -> (48.5191, 14.4431)
  line L42 (48.5191, 14.4431) -> (45.3854, 14.4431)
  line L43 (45.3854, 14.4431) -> (45.3854, 14.8224)
  line L44 (45.3854, 14.8224) -> (46.5037, 14.8224)
  spline S50 degree 2 poles (46.5037, 14.8224) (46.3748, 14.9658) (46.2047, 15.2989) (46.2047, 15.5104) knots 0 0 0 1 2 2 2
  spline S51 degree 2 poles (46.2047, 15.5104) (46.2047, 15.8921) (46.8149, 16.3297) (47.357, 16.3297) knots 0 0 0 1 2 2 2
  spline S52 degree 2 poles (47.3862, 15.9383) (46.9826, 15.9383) (46.5645, 15.6927) (46.5645, 15.4204) knots 0 0 0 1 2 2 2
  spline S53 degree 2 poles (46.5645, 15.4204) (46.5645, 15.2673) (46.7103, 14.9512) (46.8222, 14.8224) knots 0 0 0 1 2 2 2
  line L45 (46.8222, 14.8224) -> (48.1131, 14.8224)
  spline S54 degree 2 poles (48.1131, 14.8224) (48.1836, 14.9658) (48.2419, 15.1871) (48.2419, 15.3183) knots 0 0 0 1 2 2 2
  spline S55 degree 2 poles (48.2419, 15.3183) (48.2419, 15.6076) (47.8311, 15.9383) (47.3862, 15.9383) knots 0 0 0 1 2 2 2
  spline S56 degree 2 poles (48.5701, 17.7008) (48.5701, 17.1611) (47.9648, 16.5679) (47.4056, 16.5679) knots 0 0 0 1 2 2 2
  spline S57 degree 2 poles (47.4056, 16.5679) (46.8562, 16.5679) (46.2047, 17.1441) (46.2047, 17.6085) knots 0 0 0 1 2 2 2
  spline S58 degree 2 poles (46.2047, 17.6085) (46.2047, 17.8175) (46.3262, 18.1409) (46.4551, 18.26) knots 0 0 0 1 2 2 2
  spline S59 degree 2 poles (46.4551, 18.26) (46.5839, 18.3815) (46.9559, 18.5104) (47.2257, 18.5104) knots 0 0 0 1 2 2 2
  line L46 (47.2257, 18.5104) -> (47.4324, 18.5104)
  line L47 (47.4324, 18.5104) -> (47.4324, 16.9521)
  spline S60 degree 2 poles (47.4324, 16.9521) (47.8238, 16.9521) (48.2395, 17.3459) (48.2395, 17.696) knots 0 0 0 1 2 2 2
  spline S61 degree 2 poles (48.2395, 17.696) (48.2395, 17.82) (48.1836, 18.0606) (48.1398, 18.1579) knots 0 0 0 1 2 2 2
  spline S62 degree 2 poles (48.1398, 18.1579) (48.0912, 18.26) (48.0061, 18.401) (47.9672, 18.4472) knots 0 0 0 1 2 2 2
  line L48 (47.9672, 18.4472) -> (47.9672, 18.4691)
  line L49 (47.9672, 18.4691) -> (48.3805, 18.4691)
  spline S63 degree 2 poles (48.3805, 18.4691) (48.4073, 18.4034) (48.4851, 18.2041) (48.5069, 18.1263) knots 0 0 0 1 2 2 2
  spline S64 degree 2 poles (48.5069, 18.1263) (48.5385, 18.0169) (48.5701, 17.837) (48.5701, 17.7008) knots 0 0 0 1 2 2 2
  spline S65 degree 2 poles (47.1431, 18.1409) (46.9899, 18.136) (46.7663, 18.0728) (46.6909, 18.012) knots 0 0 0 1 2 2 2
  spline S66 degree 2 poles (46.6909, 18.012) (46.6058, 17.9464) (46.5159, 17.7397) (46.5159, 17.5866) knots 0 0 0 1 2 2 2
  spline S67 degree 2 poles (46.5159, 17.5866) (46.5159, 17.4358) (46.6058, 17.2243) (46.6933, 17.1368) knots 0 0 0 1 2 2 2
  spline S68 degree 2 poles (46.6933, 17.1368) (46.7833, 17.0517) (46.9996, 16.9642) (47.1431, 16.9521) knots 0 0 0 1 2 2 2
  line L50 (47.1431, 16.9521) -> (47.1431, 18.1409)
  line L51 (46.6739, 20.0882) -> (46.6739, 20.0687)
  spline S69 degree 2 poles (46.6739, 20.0687) (46.6617, 20.025) (46.6569, 19.9302) (46.6569, 19.8645) knots 0 0 0 1 2 2 2
  spline S70 degree 2 poles (46.6569, 19.8645) (46.6569, 19.7114) (46.7906, 19.4099) (46.9218, 19.2738) knots 0 0 0 1 2 2 2
  line L52 (46.9218, 19.2738) -> (48.5191, 19.2738)
  line L53 (48.5191, 19.2738) -> (48.5191, 18.8945)
  line L54 (48.5191, 18.8945) -> (46.2679, 18.8945)
  line L55 (46.2679, 18.8945) -> (46.2679, 19.2738)
  line L56 (46.2679, 19.2738) -> (46.6034, 19.2738)
  spline S71 degree 2 poles (46.6034, 19.2738) (46.4186, 19.4804) (46.2679, 19.7892) (46.2679, 19.935) knots 0 0 0 1 2 2 2
  spline S72 degree 2 poles (46.2679, 19.935) (46.2679, 19.9934) (46.2727, 20.0517) (46.28, 20.0882) knots 0 0 0 1 2 2 2
  line L57 (46.28, 20.0882) -> (46.6739, 20.0882)
  line L58 (46.6739, 21.576) -> (46.6739, 21.5566)
  spline S73 degree 2 poles (46.6739, 21.5566) (46.6617, 21.5128) (46.6569, 21.418) (46.6569, 21.3524) knots 0 0 0 1 2 2 2
  spline S74 degree 2 poles (46.6569, 21.3524) (46.6569, 21.1992) (46.7906, 20.8978) (46.9218, 20.7616) knots 0 0 0 1 2 2 2
  line L59 (46.9218, 20.7616) -> (48.5191, 20.7616)
  line L60 (48.5191, 20.7616) -> (48.5191, 20.3824)
  line L61 (48.5191, 20.3824) -> (46.2679, 20.3824)
  line L62 (46.2679, 20.3824) -> (46.2679, 20.7616)
  line L63 (46.2679, 20.7616) -> (46.6034, 20.7616)
  spline S75 degree 2 poles (46.6034, 20.7616) (46.4186, 20.9683) (46.2679, 21.277) (46.2679, 21.4229) knots 0 0 0 1 2 2 2
  spline S76 degree 2 poles (46.2679, 21.4229) (46.2679, 21.4812) (46.2727, 21.5396) (46.28, 21.576) knots 0 0 0 1 2 2 2
  line L64 (46.28, 21.576) -> (46.6739, 21.576)
  line L65 (46.2679, 23.6376) -> (49.3481, 22.4269)
  line L66 (49.3481, 22.4269) -> (49.3481, 22.0209)
  line L67 (49.3481, 22.0209) -> (48.4097, 22.4245)
  line L68 (48.4097, 22.4245) -> (46.2679, 21.6076)
  line L69 (46.2679, 21.6076) -> (46.2679, 22.0161)
  line L70 (46.2679, 22.0161) -> (47.9356, 22.6311)
  line L71 (47.9356, 22.6311) -> (46.2679, 23.2438)
  line L72 (46.2679, 23.2438) -> (46.2679, 23.6376)
  spline S77 degree 2 poles (46.4235, 27.1384) (46.618, 27.1384) (46.968, 26.9999) (47.0896, 26.8759) knots 0 0 0 1 2 2 2
  spline S78 degree 2 poles (47.0896, 26.8759) (47.2428, 26.7203) (47.4008, 26.2997) (47.4008, 25.9788) knots 0 0 0 1 2 2 2
  line L73 (47.4008, 25.9788) -> (47.4008, 25.6409)
  line L74 (47.4008, 25.6409) -> (48.5191, 25.6409)
  line L75 (48.5191, 25.6409) -> (48.5191, 25.2422)
  line L76 (48.5191, 25.2422) -> (45.5191, 25.2422)
  line L77 (45.5191, 25.2422) -> (45.5191, 25.9958)
  spline S79 degree 2 poles (45.5191, 25.9958) (45.5191, 26.2632) (45.6066, 26.6376) (45.7063, 26.7811) knots 0 0 0 1 2 2 2
  spline S80 degree 2 poles (45.7063, 26.7811) (45.8206, 26.9488) (46.1731, 27.1384) (46.4235, 27.1384) knots 0 0 0 1 2 2 2
  spline S81 degree 2 poles (46.4356, 26.7227) (46.28, 26.7227) (46.0515, 26.6157) (45.9786, 26.5063) knots 0 0 0 1 2 2 2
  spline S82 degree 2 poles (45.9786, 26.5063) (45.9154, 26.4115) (45.8643, 26.1587) (45.8643, 25.9715) knots 0 0 0 1 2 2 2
  line L78 (45.8643, 25.9715) -> (45.8643, 25.6409)
  line L79 (45.8643, 25.6409) -> (47.0604, 25.6409)
  line L80 (47.0604, 25.6409) -> (47.0604, 25.9132)
  spline S83 degree 2 poles (47.0604, 25.9132) (47.0604, 26.1563) (46.9826, 26.4553) (46.8805, 26.5525) knots 0 0 0 1 2 2 2
  spline S84 degree 2 poles (46.8805, 26.5525) (46.7906, 26.6425) (46.5791, 26.7227) (46.4356, 26.7227) knots 0 0 0 1 2 2 2
  line L81 (48.5191, 27.8751) -> (48.5191, 27.4958)
  line L82 (48.5191, 27.4958) -> (46.2679, 27.4958)
  line L83 (46.2679, 27.4958) -> (46.2679, 27.8751)
  line L84 (46.2679, 27.8751) -> (48.5191, 27.8751)
  line L85 (45.8935, 27.9018) -> (45.8935, 27.4715)
  line L86 (45.8935, 27.4715) -> (45.4996, 27.4715)
  line L87 (45.4996, 27.4715) -> (45.4996, 27.9018)
  line L88 (45.4996, 27.9018) -> (45.8935, 27.9018)
  line L89 (48.4125, 30.2277) -> (45.3625, 30.2277)
  line L90 (45.3625, 30.2277) -> (45.3625, 30.7246)
  line L91 (45.3625, 30.7246) -> (47.5222, 31.3181)
  line L92 (47.5222, 31.3181) -> (47.9744, 31.4382)
  spline S85 degree 2 poles (47.9744, 31.4382) (47.8048, 31.4806) (47.4845, 31.5701) knots 0 0 0 1 1 1
  line L93 (47.4845, 31.5701) -> (45.3625, 32.1683)
  line L94 (45.3625, 32.1683) -> (45.3625, 32.6135)
  line L95 (45.3625, 32.6135) -> (48.4125, 32.6135)
  line L96 (48.4125, 32.6135) -> (48.4125, 32.2955)
  line L97 (48.4125, 32.2955) -> (45.8618, 32.2955)
  line L98 (45.8618, 32.2955) -> (48.4125, 31.5678)
  line L99 (48.4125, 31.5678) -> (48.4125, 31.271)
  line L100 (48.4125, 31.271) -> (45.817, 30.5456)
  line L101 (45.817, 30.5456) -> (48.4125, 30.5456)
  line L102 (48.4125, 30.5456) -> (48.4125, 30.2277)
  line L103 (48.4125, 33.2023) -> (47.9862, 33.2023)
  line L104 (47.9862, 33.2023) -> (47.9862, 33.5509)
  line L105 (47.9862, 33.5509) -> (48.4125, 33.5509)
  line L106 (48.4125, 33.5509) -> (48.4125, 33.2023)
  line L107 (48.0521, 35.6093) -> (48.4125, 35.6093)
  line L108 (48.4125, 35.6093) -> (48.4125, 33.956)
  spline S86 degree 2 poles (48.4125, 33.956) (48.1934, 33.9489) (47.6517, 34.2268) (47.2843, 34.5942) knots 0 0 0 1 2 2 2
  spline S87 degree 2 poles (47.2843, 34.5942) (46.8557, 35.0229) (46.387, 35.289) (46.1868, 35.289) knots 0 0 0 1 2 2 2
  spline S88 degree 2 poles (46.1868, 35.289) (45.9536, 35.289) (45.6592, 35.0182) (45.6592, 34.818) knots 0 0 0 1 2 2 2
  spline S89 degree 2 poles (45.6592, 34.818) (45.6592, 34.6036) (45.9772, 34.3304) (46.2739, 34.3304) knots 0 0 0 1 2 2 2
  line L109 (46.2739, 34.3304) -> (46.2339, 34.0148)
  spline S90 degree 2 poles (46.2339, 34.0148) (45.7935, 34.0478) (45.3507, 34.4788) (45.3507, 34.8297) knots 0 0 0 1 2 2 2
  spline S91 degree 2 poles (45.3507, 34.8297) (45.3507, 35.2113) (45.8665, 35.6046) (46.1939, 35.6046) knots 0 0 0 1 2 2 2
  spline S92 degree 2 poles (46.1939, 35.6046) (46.4859, 35.6046) (47.0205, 35.2961) (47.4657, 34.8674) knots 0 0 0 1 2 2 2
  spline S93 degree 2 poles (47.4657, 34.8674) (47.7459, 34.5919) (47.9508, 34.4317) (48.0521, 34.3822) knots 0 0 0 1 2 2 2
  line L110 (48.0521, 34.3822) -> (48.0521, 35.6093)
  line L111 (48.4125, 37.0366) -> (45.3625, 37.0366)
  line L112 (45.3625, 37.0366) -> (45.3625, 37.3663)
  line L113 (45.3625, 37.3663) -> (46.6154, 37.3663)
  line L114 (46.6154, 37.3663) -> (46.6154, 38.6687)
  line L115 (46.6154, 38.6687) -> (45.3625, 38.6687)
  line L116 (45.3625, 38.6687) -> (45.3625, 38.9985)
  line L117 (45.3625, 38.9985) -> (48.4125, 38.9985)
  line L118 (48.4125, 38.9985) -> (48.4125, 38.6687)
  line L119 (48.4125, 38.6687) -> (46.9758, 38.6687)
  line L120 (46.9758, 38.6687) -> (46.9758, 37.3663)
  line L121 (46.9758, 37.3663) -> (48.4125, 37.3663)
  line L122 (48.4125, 37.3663) -> (48.4125, 37.0366)
  line L123 (48.4125, 39.2858) -> (45.3625, 40.2467)
  line L124 (45.3625, 40.2467) -> (45.3625, 40.6047)
  line L125 (45.3625, 40.6047) -> (48.4125, 41.6269)
  line L126 (48.4125, 41.6269) -> (48.4125, 41.2477)
  line L127 (48.4125, 41.2477) -> (47.4892, 40.958)
  line L128 (47.4892, 40.958) -> (47.4892, 39.9076)
  line L129 (47.4892, 39.9076) -> (48.4125, 39.6367)
  line L130 (48.4125, 39.6367) -> (48.4125, 39.2858)
  line L131 (47.1595, 40.0041) -> (47.1595, 40.8544)
  line L132 (47.1595, 40.8544) -> (46.314, 40.5953)
  spline S94 degree 2 poles (46.314, 40.5953) (45.9254, 40.4728) (45.6828, 40.4187) knots 0 0 0 1 1 1
  spline S95 degree 2 poles (45.6828, 40.4187) (45.9772, 40.3692) (46.2645, 40.2821) knots 0 0 0 1 1 1
  line L133 (46.2645, 40.2821) -> (47.1595, 40.0041)
  line L134 (48.4125, 42.5313) -> (45.7228, 42.5313)
  line L135 (45.7228, 42.5313) -> (45.7228, 41.707)
  line L136 (45.7228, 41.707) -> (45.3625, 41.707)
  line L137 (45.3625, 41.707) -> (45.3625, 43.69)
  line L138 (45.3625, 43.69) -> (45.7228, 43.69)
  line L139 (45.7228, 43.69) -> (45.7228, 42.861)
  line L140 (45.7228, 42.861) -> (48.4125, 42.861)
  line L141 (48.4125, 42.861) -> (48.4125, 42.5313)
  line L142 (47.9202, 44.6251) -> (47.0841, 44.6251)
  line L143 (47.0841, 44.6251) -> (47.0841, 43.9444)
  line L144 (47.0841, 43.9444) -> (46.7356, 43.9444)
  line L145 (46.7356, 43.9444) -> (46.7356, 44.6251)
  line L146 (46.7356, 44.6251) -> (45.9065, 44.6251)
  line L147 (45.9065, 44.6251) -> (45.9065, 44.9171)
  line L148 (45.9065, 44.9171) -> (46.7356, 44.9171)
  line L149 (46.7356, 44.9171) -> (46.7356, 45.5978)
  line L150 (46.7356, 45.5978) -> (47.0841, 45.5978)
  line L151 (47.0841, 45.5978) -> (47.0841, 44.9171)
  line L152 (47.0841, 44.9171) -> (47.9202, 44.9171)
  line L153 (47.9202, 44.9171) -> (47.9202, 44.6251)
  line L154 (52.6404, 38.6295) -> (50.1004, 38.6295)
  line L155 (50.1004, 38.6295) -> (50.1004, 39.0433)
  line L156 (50.1004, 39.0433) -> (51.899, 39.5376)
  line L157 (51.899, 39.5376) -> (52.2755, 39.6376)
  spline S96 degree 2 poles (52.2755, 39.6376) (52.1343, 39.673) (51.8676, 39.7475) knots 0 0 0 1 1 1
  line L158 (51.8676, 39.7475) -> (50.1004, 40.2457)
  line L159 (50.1004, 40.2457) -> (50.1004, 40.6164)
  line L160 (50.1004, 40.6164) -> (52.6404, 40.6164)